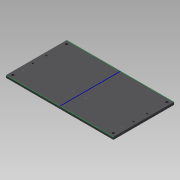
# Autodesk Inventor part: 基本板
Saved by Autodesk Inventor 2017 (Build 210142000, 142)
## iProperties
Part Number: 基本板
Material: アルミニウム 5052
Document SubType Name: Modeling
Designer: HISAAKI
Density: 2.68 g/cm^3
Appearance: サテン - ブラシ仕上げ 重厚
Mass: 99.9866 g
Surface Area: 243.169 cm^2
Volume: 37.3084 cm^3
Author: HISAAKI
Autodesk Inventor part; units mm, degrees
ref_plane "YZ Plane" through (0, 0, 0) normal (1, 0, 0) x (0, 1, 0)
ref_plane "XZ Plane" through (0, 0, 0) normal (0, 1, 0) x (-1, 0, 0)
ref_plane "XY Plane" through (0, 0, 0) normal (0, 0, 1) x (1, 0, 0)
sketch "スケッチ1" plane through (0, 0, 0) normal (0, 1, 0) x (-1, 0, 0)
  line L0 (0, 0) -> (80, 0)
  line L1 (80, 0) -> (80, -142)
  line L2 (80, -142) -> (0, -142)
  line L3 (0, -142) -> (0, 0)
  dimension "d0" = 80
  dimension "d1" = 142
  constraints: 8 end point, 2 parallel, 1 horizontal, 1 perpendicular
  measures "d0" distance of L1.end L2.end
  measures "d1" distance of L0.end L1.end
extrude "押し出し1" add sketch "スケッチ1" along normal blind 3.3
hole "穴1" at (-75.5, 3.3, -4.5) direction (0, -1, 0) diameter 3.4 end through all
hole "穴2" at (-4.5, 3.3, -4.5) direction (0, -1, 0) diameter 3.4 end through all
hole "穴3" at (-4.5, 3.3, -137.5) direction (0, -1, 0) diameter 3.4 end through all
hole "穴4" at (-75.5, 3.3, -137.5) direction (0, -1, 0) diameter 3.4 end through all
hole "穴5" at (-49, 3.3, -137.75) direction (0, -1, 0) diameter 2.4 end through all
hole "穴6" at (-31, 3.3, -137.75) direction (0, -1, 0) diameter 2.4 end through all
hole "穴7" at (-31, 3.3, -4.25) direction (0, -1, 0) diameter 2.4 end through all
hole "穴8" at (-49, 3.3, -4.25) direction (0, -1, 0) diameter 2.4 end through all
hole "穴9" at (-7, 0, -71) direction (0, 1, 0) diameter 2.4 end through all
hole "穴10" at (-23, 0, -71) direction (0, 1, 0) diameter 2.4 end through all
sketch "スケッチ3" plane through (0, 3.3, 0) normal (0, 1, 0) x (1, 0, 0)
  line L0 (0, 0) -> (0, 142) projected
  line L1 (0, 71) -> (-80, 71)
  line L2 (-80, 142) -> (-80, 0) projected
  constraints: 2 end point, 2 midpoint
